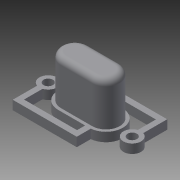
# Autodesk Inventor part: button
Saved by Autodesk Inventor 2014 (Build 180170000, 170)
## iProperties
Created: 2013-09-15
Part Number: button
Material: Generic
Document SubType Name: Modeling
Designer: stephen
Density: 1 g/cm^3
Appearance: Default
Author: stephen
Autodesk Inventor part; units mm, degrees
ref_plane "YZ Plane" through (0, 0, 0) normal (1, 0, 0) x (0, 1, 0)
ref_plane "XZ Plane" through (0, 0, 0) normal (0, 1, 0) x (-1, 0, 0)
ref_plane "XY Plane" through (0, 0, 0) normal (0, 0, 1) x (1, 0, 0)
sketch "Sketch1" plane through (0, 0, 0) normal (0, 0, 1) x (1, 0, 0)
  line L0 (4.9374, 6.4254) -> (10.2374, 6.4254) construction
  line L1 (4.9374, 4.0754) -> (10.2374, 4.0754)
  line L2 (10.2374, 8.7754) -> (4.9374, 8.7754)
  arc A0 (4.9374, 8.7754) -> (4.9374, 4.0754) centre (4.9374, 6.4254) ccw
  arc A1 (10.2374, 4.0754) -> (10.2374, 8.7754) centre (10.2374, 6.4254) ccw
  point P0 (0, 0)
  point P1 (7.5874, 6.4254)
  dimension "d0" = 10
  dimension "d1" = 4.7
  constraints: 8 end point, 4 point on circle, 4 tangent, 2 centre point, 1 horizontal, 1 midpoint, 1 parallel
  measures "d1" distance between parallel lines of L1 L2
extrude "Extrusion1" add sketch "Sketch1" along normal blind 7.3
fillet "Fillet1" radius 1 4 edges at (7.5874, 8.7754, 7.3) (2.5874, 6.4254, 7.3) (7.5874, 4.0754, 7.3) (12.5874, 6.4254, 7.3)
sketch "Sketch2" plane through (0, 0, 0) normal (0, 0, -1) x (-1, 0, 0)
  line L0 (-4.9374, 4.0754) -> (-10.2374, 4.0754) projected
  arc A0 (-4.9374, 4.0754) -> (-4.9374, 8.7754) centre (-4.9374, 6.4254) ccw projected
  line L1 (-10.2374, 8.7754) -> (-4.9374, 8.7754) projected
  arc A1 (-10.2374, 8.7754) -> (-10.2374, 4.0754) centre (-10.2374, 6.4254) ccw projected
  line L2 (-10.2374, 6.4254) -> (-4.9374, 6.4254) construction
  line L3 (-10.2374, 3.5754) -> (-4.9374, 3.5754)
  line L4 (-4.9374, 9.2754) -> (-10.2374, 9.2754)
  arc A2 (-10.2374, 9.2754) -> (-10.2374, 3.5754) centre (-10.2374, 6.4254) ccw
  arc A3 (-4.9374, 3.5754) -> (-4.9374, 9.2754) centre (-4.9374, 6.4254) ccw
  point P0 (0, 0)
  point P1 (-7.5874, 6.4254)
  dimension "d5" = 0.5
  constraints: 8 end point, 4 point on circle, 4 tangent, 2 centre point, 2 parallel, 1 midpoint
  measures "d5" distance between parallel lines of L3 L0
extrude "Extrusion2" add sketch "Sketch2" along normal blind 1.54
sketch "Sketch3" plane through (0, 0, 0) normal (0, 0, -1) x (-1, 0, 0)
  line L0 (-4.9374, 4.0754) -> (-10.2374, 4.0754) projected
  arc A0 (-4.9374, 4.0754) -> (-4.9374, 8.7754) centre (-4.9374, 6.4254) ccw projected
  line L1 (-10.2374, 8.7754) -> (-4.9374, 8.7754) projected
  arc A1 (-10.2374, 8.7754) -> (-10.2374, 4.0754) centre (-10.2374, 6.4254) ccw projected
  line L2 (-10.2374, 6.4254) -> (-4.9374, 6.4254) construction
  line L3 (-10.2374, 3.6254) -> (-4.9374, 3.6254)
  line L4 (-4.9374, 9.2254) -> (-10.2374, 9.2254)
  arc A2 (-10.2374, 9.2254) -> (-10.2374, 3.6254) centre (-10.2374, 6.4254) ccw
  arc A3 (-4.9374, 3.6254) -> (-4.9374, 9.2254) centre (-4.9374, 6.4254) ccw
  point P0 (0, 0)
  point P1 (-7.5874, 6.4254)
  constraints: 8 end point, 4 point on circle, 4 tangent, 2 centre point, 2 parallel, 1 midpoint
extrude "Extrusion3" add sketch "Sketch3" along normal blind 1.54 contours L0 A1 L1 A0
sketch "Sketch4" plane through (0, 0, -1.54) normal (0, 0, -1) x (-1, 0, 0)
  line L0 (-4.9374, 9.2754) -> (-10.2374, 9.2754) projected
  arc A0 (-10.2374, 9.2754) -> (-10.2374, 3.5754) centre (-10.2374, 6.4254) ccw projected
  line L1 (-10.2374, 6.4254) -> (-7.6274, 6.4254)
  circle A1 centre (-7.6274, 6.4254) radius 1.3
  point P0 (0, 0)
  dimension "d10" = 2.61
  dimension "d11" = 2.6
  constraints: 2 end point, 1 centre point, 1 coincident, 1 parallel
  measures "d10" distance of L1.start L1.end
  measures "d11" diameter of A1
extrude "Extrusion4" cut sketch "Sketch4" against normal blind 2.96
sketch "Sketch5" plane through (0, 0, -1.54) normal (0, 0, -1) x (-1, 0, 0)
  arc A0 (-4.9374, 3.5754) -> (-4.9374, 9.2754) centre (-4.9374, 6.4254) ccw projected
  line L0 (-4.9374, 9.2754) -> (-10.2374, 9.2754) projected
  circle A1 centre (-15.1574, 5.9754) radius 0.8
  arc A2 (-15.6111, 7.4051) -> (-14.6795, 7.3972) centre (-15.1574, 5.9754) ccw
  line L1 (-15.6111, 8.031) -> (-15.6271, 8.031)
  line L2 (-15.6111, 7.4051) -> (-15.6111, 10.4765)
  line L3 (-4.6841, 10.5736) -> (-4.6841, 9.2641)
  line L4 (-14.6795, 7.3972) -> (-14.6795, 9.4832)
  line L5 (-5.6379, 9.578) -> (-5.6379, 9.2754)
  line L6 (-10.2374, 3.5754) -> (-4.9374, 3.5754) projected
  line L7 (-15.6111, 10.4765) -> (-15.6111, 11.4765)
  line L8 (-15.6111, 11.4765) -> (-4.6841, 11.4765)
  line L9 (-4.6841, 11.4765) -> (-4.6841, 10.2108)
  line L10 (-14.6795, 9.4832) -> (-14.6795, 10.4832)
  line L11 (-14.6795, 10.4832) -> (-5.6379, 10.4832)
  line L12 (-5.6379, 10.4832) -> (-5.6379, 9.578)
  point P0 (0, 0)
  dimension "d15" = 1.6
  dimension "d34" = 1
  dimension "d39" = 0.7
  constraints: 22 end point, 3 parallel, 3 point on circle, 3 point on line, 2 centre point, 2 perpendicular, 1 coincident
  measures "d15" diameter of A1
  measures "d34" distance of L2.end L7.end
  measures "d39" radial gap between concentric circles of A2 A1
extrude "Extrusion5" add sketch "Sketch5" against normal blind 1.54
sketch "Sketch6" plane through (0, 0, -1.54) normal (0, 0, -1) x (-1, 0, 0)
  line L0 (-10.2374, 3.5754) -> (-4.9374, 3.5754) projected
  arc A0 (-10.2374, 9.2754) -> (-10.2374, 3.5754) centre (-10.2374, 6.4254) ccw projected
  circle A1 centre (-0.0485, 6.7803) radius 0.8
  arc A2 (0.4175, 5.3545) -> (-0.5144, 5.3545) centre (-0.0485, 6.7803) ccw
  line L1 (0.4175, 5.3545) -> (0.4175, 2.2034)
  line L2 (-0.5144, 3.7394) -> (-0.5144, 5.3545)
  line L3 (-0.5144, 3.7394) -> (-0.5144, 3.1974)
  line L4 (-10.4904, 2.2016) -> (-10.4904, 3.5866)
  line L5 (-9.5364, 3.1974) -> (-9.5364, 3.5754)
  line L6 (-5.6379, 10.4832) -> (-5.6379, 9.2754) projected
  line L7 (0.4175, 2.2034) -> (0.4175, 1.2016)
  line L8 (0.4175, 1.2016) -> (-10.4904, 1.2016)
  line L9 (-10.4904, 1.2016) -> (-10.4904, 2.2016)
  line L10 (-0.5144, 3.1974) -> (-0.5144, 2.1974)
  line L11 (-0.5144, 2.1974) -> (-9.5364, 2.1974)
  line L12 (-9.5364, 2.1974) -> (-9.5364, 3.1974)
  point P0 (0, 0)
  point P1 (-1.5346, 6.984)
  dimension "d22" = 1.6
  dimension "d37" = 1
  dimension "d40" = 0.7
  constraints: 22 end point, 4 parallel, 4 point on circle, 3 perpendicular, 2 centre point, 1 coincident, 1 point on line
  measures "d22" diameter of A1
  measures "d37" distance of L3.end L10.end
  measures "d40" radial gap between concentric circles of A2 A1
extrude "Extrusion6" add sketch "Sketch6" against normal blind 1.54
body "Solid1"
